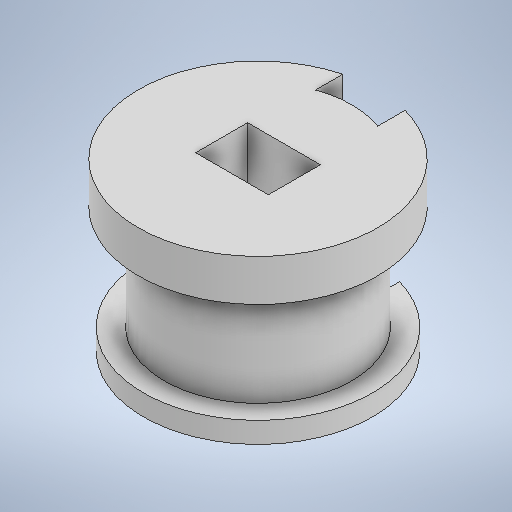
# Autodesk Inventor part: 圓形同心線圈內
Saved by Autodesk Inventor 2025.2 (Build 292293000, 293)
## iProperties
Created: 2025-07-25
Part Number: 圓形同心線圈內
Material: 一般
Document SubType Name: Modeling
Designer: 123
Density: 1 g/cm^3
Appearance: 預設
Author: 123
Autodesk Inventor part; units mm, degrees
ref_plane "YZ Plane" through (0, 0, 0) normal (1, 0, 0) x (0, 1, 0)
ref_plane "XZ Plane" through (0, 0, 0) normal (0, 1, 0) x (-1, 0, 0)
ref_plane "XY Plane" through (0, 0, 0) normal (0, 0, 1) x (1, 0, 0)
sketch "草圖1" plane through (0, 0, 0) normal (0, 1, 0) x (-1, 0, 0)
  circle A0 centre (0, 0) radius 5.75
  dimension "d0" = 11.5
  constraints: 1 centre point, 1 coincident
  measures "d0" diameter of A0
extrude "擠出1" add sketch "草圖1" along normal blind 2
sketch "草圖2" plane through (0, 0, 0) normal (0, -1, 0) x (1, 0, 0)
  circle A0 centre (0, 0) radius 4.5
  dimension "d3" = 9
  constraints: 1 centre point, 1 coincident
  measures "d3" diameter of A0
extrude "擠出2" add sketch "草圖2" along normal blind 5
sketch "草圖3" plane through (0, -5, 0) normal (0, -1, 0) x (1, 0, 0)
  circle A0 centre (0, 0) radius 5.5
  constraints: 1 centre point, 1 coincident
extrude "擠出3" add sketch "草圖3" along normal blind 1
sketch "草圖4" plane through (0, 2, 0) normal (0, 1, 0) x (1, 0, 0)
  line L0 (-1.75, 1.25) -> (1.75, 1.25)
  line L1 (1.75, 1.25) -> (1.75, -1.25)
  line L2 (1.75, -1.25) -> (-1.75, -1.25)
  line L3 (-1.75, -1.25) -> (-1.75, 1.25)
  line L4 (-1.75, 1.25) -> (1.75, -1.25) construction
  line L5 (1.75, 1.25) -> (-1.75, -1.25) construction
  point P0 (0, 0)
  dimension "d8" = 2.5
  dimension "d9" = 3.5
  constraints: 12 end point, 2 midpoint, 2 parallel, 1 horizontal, 1 perpendicular
  measures "d8" distance of L0.end L1.end
  measures "d9" distance of L0.start L0.end
extrude "擠出4" cut sketch "草圖4" against normal through all
sketch "草圖5" plane through (0, 2, 0) normal (0, 1, 0) x (1, 0, 0)
  line L0 (-1.4797, 3) -> (1.5203, 3)
  line L1 (1.5203, 3) -> (1.5203, 6)
  line L2 (1.5203, 6) -> (-1.4797, 6)
  line L3 (-1.4797, 6) -> (-1.4797, 3)
  circle A0 centre (0, 0) radius 4.5 projected
  line L4 (-1.4797, 3) -> (1.5203, 6) construction
  line L5 (1.5203, 3) -> (-1.4797, 6) construction
  point P0 (0.0203, 4.5)
  point P1 (-1.4797, 4.2497)
  point P2 (1.5203, 4.2354)
  dimension "d12" = 3
  dimension "d15" = 3
  constraints: 12 end point, 2 midpoint, 2 parallel, 1 horizontal, 1 perpendicular, 2 other
  measures "d12" distance of L2.end L0.start
  measures "d15" distance of L1.end L2.end
extrude "擠出5" cut sketch "草圖5" against normal through all contours L3 L2 L1 A0
